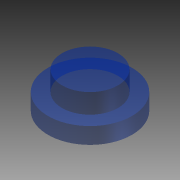
# Autodesk Inventor part: nivel
Saved by Autodesk Inventor 2016 (Build 200138000, 138)
## iProperties
Created: 2013-07-10
Part Number: nivel
Material: Generic
Document SubType Name: Modeling
Designer: Luis
Density: 1 g/cm^3
Appearance: Clear - Blue
Author: Luis
Autodesk Inventor part; units mm, degrees
ref_plane "YZ Plane" through (0, 0, 0) normal (1, 0, 0) x (0, 1, 0)
ref_plane "XZ Plane" through (0, 0, 0) normal (0, 1, 0) x (-1, 0, 0)
ref_plane "XY Plane" through (0, 0, 0) normal (0, 0, 1) x (1, 0, 0)
sketch "Sketch1" plane through (0, 0, 0) normal (0, 0, 1) x (1, 0, 0)
  circle A0 centre (0, 0) radius 6
  circle A1 centre (0, 0) radius 9
  point P0 (14, 6.5)
  constraints: 2 centre point
extrude "Extrusion1" add sketch "Sketch1" along normal blind 3.5
extrude "Extrusion2" add sketch "Sketch1" along normal blind 7.7 contours A0
body "Solid1"
